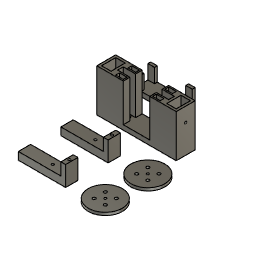
final v1 (Autodesk Fusion 360 design; units mm, degrees)
Autodesk Fusion 360 part; units mm, degrees
note: some values were not read from the file. Chosen so that the rebuilt part matches the saved one: which face or edge a step refers to; how an offset face is resized. Set by a fixed rule: which sketch regions a step uses.
sketch "Sketch1" plane through (0, 0, 0) normal (0, 0, 1) x (1, 0, 0)
  line L0 (0, 0) -> (84, 0)
  line L1 (84, 0) -> (84, 20)
  line L2 (84, 20) -> (0, 20)
  line L3 (0, 20) -> (0, 0)
  line L4 (0, 0) -> (0, 10)
  line L5 (0, 10) -> (84, 10) construction
  line L6 (42, 0) -> (42, 20) construction
  line L7 (42, 10) -> (60, 10) construction
  line L8 (42, 10) -> (24, 10) construction
  circle A0 centre (60, 10) radius 1.5
  circle A1 centre (24, 10) radius 1.5
  line L9 (79, 5) -> (79, 15)
  line L10 (5, 15) -> (5, 5)
  line L11 (5, 15) -> (10, 15)
  line L12 (10, 15) -> (10, 5)
  line L13 (79, 15) -> (74, 15)
  line L14 (74, 15) -> (74, 5)
  line L15 (79, 15) -> (74, 15)
  line L16 (10, 15) -> (5, 15)
  line L17 (5, 5) -> (10, 5)
  line L18 (74, 5) -> (79, 5)
  line L19 (0, 20) -> (15, 20)
  line L20 (15, 10) -> (15, 20)
  line L21 (84, 20) -> (69, 20)
  line L22 (69, 20) -> (69, 0)
  line L23 (15, 10) -> (15, 0)
  line L24 (12.5, 17.5) -> (2.5, 17.5)
  line L25 (2.5, 17.5) -> (2.5, 2.5)
  line L26 (2.5, 2.5) -> (12.5, 2.5)
  line L27 (12.5, 17.5) -> (12.5, 2.5)
  line L28 (71.5, 17.5) -> (71.5, 2.5)
  line L29 (71.5, 2.5) -> (81.5, 2.5)
  line L30 (81.5, 2.5) -> (81.5, 17.5)
  line L31 (81.5, 17.5) -> (71.5, 17.5)
  line L32 (0, 20) -> (0, 40) construction
  line L33 (0, 40) -> (47, 40)
  line L34 (47, 40) -> (47, 57)
  line L35 (47, 57) -> (0, 57)
  line L36 (0, 57) -> (0, 40)
  line L37 (0, 57) -> (7, 57)
  line L38 (7, 57) -> (7, 54)
  line L39 (7, 54) -> (0, 54)
  line L40 (0, 54) -> (0, 57)
  line L41 (0, 40) -> (0, 48.5)
  line L42 (47, 48.5) -> (0, 48.5)
  line L43 (0, 40) -> (7, 40)
  line L44 (7, 40) -> (7, 43)
  line L45 (7, 43) -> (0, 43)
  line L46 (0, 43) -> (0, 40)
  line L47 (47, 57) -> (40, 57)
  line L48 (40, 57) -> (40, 54)
  line L49 (40, 54) -> (47, 54)
  line L50 (47, 54) -> (47, 57)
  line L51 (47, 40) -> (40, 40)
  line L52 (40, 40) -> (40, 43)
  line L53 (40, 43) -> (47, 43)
  line L54 (47, 43) -> (47, 40)
  dimension "d1" = 84
  dimension "d2" = 20
  dimension "d6" = 3
  dimension "d7" = 3
  dimension "d9" = 5
  dimension "d10" = 5
  dimension "d31" = 2.5
  dimension "d32" = 2.5
  dimension "d96" = 47
  dimension "d97" = 17
  dimension "d98" = 3
  dimension "d99" = 7
  dimension "d100" = 3
  dimension "d101" = 7
  dimension "d102" = 3
  dimension "d103" = 7
  dimension "d104" = 3
  dimension "d105" = 7
  constraint coincident L0.start L3.end
  constraint horizontal L0
  constraint perpendicular L0 L1
  constraint perpendicular L1 L2
  constraint perpendicular L0 L3
  constraint midpoint L3 L4.end
  constraint midpoint L1 L5.end
  constraint midpoint L2 L6.end
  constraint perpendicular L2 L6
  constraint coincident L0 L6.start
  constraint midpoint L6 L7.start
  constraint perpendicular L6 L7
  constraint perpendicular L6 L8
  constraint coincident L7.end A0.centre
  constraint coincident L8.end A1.centre
  constraint perpendicular L10 L11
  constraint perpendicular L12 L17
  constraint perpendicular L9 L13
  constraint coincident L14.end L17
  constraint perpendicular L14 L17
  constraint collinear L15 L16
  constraint collinear L17 L18
  constraint coincident L2 L19.end
  constraint perpendicular L2 L20
  constraint coincident L2 L21.end
  constraint coincident L0 L22.end
  constraint perpendicular L0 L22
  constraint coincident L5 L20.start
  constraint coincident L0 L23.end
  constraint perpendicular L0 L23
  constraint perpendicular L19 L32
  constraint horizontal L33
  constraint vertical L34
  constraint horizontal L35
  constraint vertical L36
  constraint horizontal L37
  constraint vertical L38
  constraint horizontal L39
  constraint vertical L40
  constraint midpoint L36 L41.end
  constraint midpoint L34 L42.start
  constraint horizontal L43
  constraint vertical L44
  constraint horizontal L45
  constraint vertical L46
  constraint horizontal L47
  constraint vertical L48
  constraint horizontal L49
  constraint vertical L50
  constraint horizontal L51
  constraint vertical L52
  constraint horizontal L53
  constraint vertical L54
  measures "d1" distance of L0.start L0.end
  measures "d2" distance of L0.end L1.end
  measures "d6" diameter of A0
  measures "d7" diameter of A1
  measures "d9" distance of L10.start L11.end
  measures "d10" distance of L9.end L13.end
  measures "d96" distance of L32.end L33.end
  measures "d97" distance of L33.end L34.end
  measures "d98" distance of L37.end L38.end
  measures "d99" distance of L38.end L39.end
  measures "d100" distance of L43.end L44.end
  measures "d101" distance of L44.end L45.end
  measures "d102" distance of L47.end L48.end
  measures "d103" distance of L48.end L49.end
  measures "d104" distance of L51.end L52.end
  measures "d105" distance of L52.end L53.end
extrude "Extrude1" add sketch "Sketch1" along normal blind 5 contours L0 L2 L20 L22 L23 makes body 1
extrude "Extrude2" add sketch "Sketch1" along normal blind 45 contours L0 L2 L3 L4 L19 L20 L23 | L24 L25 L26 L27 bodies 1
extrude "Extrude3" add sketch "Sketch1" along normal blind 45 contours L0 L1 L2 L21 L22 | L28 L29 L30 L31 bodies 1
sketch "Sketch2" plane through (0, 0, 5) normal (0, 0, 1) x (-1, 0, 0)
  circle A0 centre (-24, -10) radius 1.5
  circle A1 centre (-60, -10) radius 1.5
  line L0 (-69, -20) -> (-15, -20)
  line L1 (-15, -20) -> (-15, 0)
  line L2 (-15, 0) -> (-69, 0)
  line L3 (-69, 0) -> (-69, -20)
  line L4 (-42, -10) -> (-56, -10)
  line L5 (-56, -13) -> (-56, -20)
  line L6 (-56, -7) -> (-56, 0)
  line L7 (-42, -10) -> (-28, -10)
  line L8 (-28, -7) -> (-28, 0)
  line L9 (-28, -13) -> (-28, -20)
  line L10 (-26, -13) -> (-26, -20)
  line L11 (-26, -7) -> (-26, 0)
  line L12 (-58, -13) -> (-58, -20)
  line L13 (-58, -7) -> (-58, 0)
  line L14 (-26, -20) -> (-26, -13)
  line L15 (-26, -20) -> (-26, -13)
  line L16 (-28, -13) -> (-26, -13)
  line L17 (-56, -20) -> (-56, -13)
  line L18 (-58, -13) -> (-56, -13)
  line L19 (-26, 0) -> (-26, -7)
  line L20 (-28, -7) -> (-26, -7)
  line L21 (-56, 0) -> (-56, -7)
  line L22 (-58, -7) -> (-56, -7)
  dimension "d18" = -2
  dimension "d20" = 2
  dimension "d22" = 14
  constraint horizontal L4
  constraint coincident L0 L5.end
  constraint perpendicular L0 L5
  constraint coincident L2 L6.end
  constraint perpendicular L2 L6
  constraint parallel L4 L7
  constraint coincident L2 L8.end
  constraint perpendicular L2 L8
  constraint coincident L0 L9.end
  constraint perpendicular L0 L9
  constraint coincident L10 L14.end
  constraint perpendicular L7 L14
  constraint perpendicular L15 L16
  constraint coincident L12 L18.start
  constraint perpendicular L5 L18
  constraint perpendicular L19 L20
  constraint perpendicular L6 L22
  measures "d22" distance of L4.start L7.end
extrude "Extrude4" add sketch "Sketch2" along normal blind 14 contours L0 L9 L10 L14 L15 L16 bodies 1
extrude "Extrude5" cut 1 faces at (27.3333, 15.3333, 19) along direction (0, 0, -1) blind 14 on bodies 1 bodies 1
extrude "Extrude6" cut 1 faces at (36.1113, 2.8459, 0) along direction (0, 0, -1) blind 14 on bodies 1 bodies 1
extrude "Extrude7" add sketch "Sketch2" along normal blind 20 contours L0 L5 L12 L17 L18 | L2 L6 L13 L21 L22 | L0 L9 L10 L14 L15 L16 | L2 L8 L11 L19 L20 bodies 1
extrude "Extrude8" cut sketch "Sketch1" along normal blind 55 contours L24 L25 L26 L27 bodies 1
extrude "Extrude9" cut sketch "Sketch1" along normal blind 53 contours L28 L29 L30 L31 bodies 1
sketch "Sketch4" plane through (0, 0, 0) normal (1, 0, 0) x (0, 1, 0)
  line L0 (0, 0) -> (-20, 0) construction
  line L1 (-20, 0) -> (-28, 0)
  line L2 (-28, 0) -> (-28, 13)
  line L3 (-28, 13) -> (-20, 13)
  line L4 (-20, 13) -> (-20, 0)
  dimension "d40" = 20
  dimension "d41" = 8
  dimension "d42" = 13
  constraint coincident L0.start origin
  constraint horizontal L0
  constraint horizontal L1
  constraint vertical L2
  constraint horizontal L3
  constraint vertical L4
  measures "d40" distance of L0.start L0.end
  measures "d41" distance of L0.end L1.end
  measures "d42" distance of L1.end L2.end
extrude "Extrude10" add sketch "Sketch4" along normal blind 50 separate body makes body 2
sketch "Sketch5" plane through (0, -28, 0) normal (0, -1, 0) x (1, 0, 0)
  line L0 (0, 13) -> (0, 0)
  line L1 (0, 0) -> (50, 0)
  line L2 (50, 0) -> (50, 13)
  line L3 (50, 13) -> (0, 13)
  line L4 (50, 13) -> (45, 13)
  line L5 (45, 13) -> (45, 0)
  dimension "d45" = 5
  constraint coincident L2.end L3.start
  constraint perpendicular L2 L4
  constraint coincident L1 L5.end
  constraint perpendicular L1 L5
  measures "d45" distance of L2.end L4.end
extrude "Extrude11" add sketch "Sketch5" along normal blind 15 contours L1 L2 L3 L4 L5 bodies 2
sketch "Sketch6" plane through (0, 0, 0) normal (0, 0, 1) x (1, 0, 0)
  circle A0 centre (84, -30) radius 18
  line L0 (88.7553, -25.2447) -> (89.8867, -24.1133)
  line L1 (88.7553, -34.7553) -> (89.8867, -35.8867)
  line L2 (79.2447, -25.2447) -> (78.1133, -24.1133)
  line L3 (79.2447, -34.7553) -> (78.1133, -35.8867)
  circle A1 centre (89.8867, -24.1133) radius 1.6
  circle A2 centre (78.1133, -24.1133) radius 1.6
  circle A3 centre (89.8867, -35.8867) radius 1.6
  circle A4 centre (78.1133, -35.8867) radius 1.6
  arc A5 (79.3482, -23.0959) -> (77.0959, -25.3482) centre (84, -30) ccw
  arc A6 (77.0959, -34.6518) -> (78.1133, -35.8867) centre (84, -30) ccw
  arc A7 (88.6518, -36.9041) -> (90.9041, -34.6518) centre (84, -30) ccw
  arc A8 (90.9041, -25.3482) -> (88.6518, -23.0959) centre (84, -30) ccw
  circle A9 centre (84, -30) radius 1.5
  dimension "d49" = 36
  dimension "d50" = 16.65
  dimension "d51" = 3.2
  dimension "d52" = 3.2
  dimension "d53" = 3.2
  dimension "d54" = 3.2
  dimension "d57" = 3
  constraint concentric A0 A5
  constraint coincident L1.end A5
  constraint perpendicular L0 L1
  constraint perpendicular L0 L2
  constraint perpendicular L2 L3
  constraint coincident L3.end A5
  constraint coincident L0.end A5
  constraint coincident L2.end A5
  constraint coincident L0.end A1.centre
  constraint coincident L2.end A2.centre
  constraint coincident L1.end A3.centre
  constraint coincident L3.end A4.centre
  constraint coincident A1 A8.end
  constraint coincident A2 A5.start
  constraint coincident A2 A5.end
  constraint coincident A4 A6.start
  constraint concentric A5 A6
  constraint concentric A6 A7
  constraint coincident A3 A7.start
  constraint coincident A3 A7.end
  constraint coincident A1 A8.start
  constraint concentric A7 A8
  constraint coincident A3 L1.start
  constraint coincident A4 L3.start
  constraint coincident A1 L0.start
  constraint coincident A2 L2.start
  constraint concentric A6 A9
  measures "d49" diameter of A0
  measures "d50" diameter of A5
  measures "d51" diameter of A1
  measures "d52" diameter of A2
  measures "d53" diameter of A3
  measures "d54" diameter of A4
  measures "d57" diameter of A9
extrude "Extrude12" add sketch "Sketch6" along normal blind 3 separate body contours A0 | A9 makes body 3
sketch "Sketch7" plane through (0, 0, 3) normal (0, 0, 1) x (-1, 0, 0)
  circle A0 centre (-78.1133, 35.8867) radius 1.6
  circle A1 centre (-89.8867, 35.8867) radius 1.6
  circle A2 centre (-78.1133, 24.1133) radius 1.6
  circle A3 centre (-89.8867, 24.1133) radius 1.6
  circle A4 centre (-84, 30) radius 18
  circle A5 centre (-84, 30) radius 1.5
  dimension "d58" = 3
  constraint concentric A4 A5
  measures "d58" diameter of A5
extrude "Extrude13" cut sketch "Sketch7" against normal blind 11 contours A5 bodies 3
thread "Thread1" "ISO Metric profile 3.0 M3x0.5 6H" major diameter 3.086 minor diameter 2.529 pitch 0.5 angle 60 resizes the face on face at (82.8043, -30.9057, 1) on bodies 3
sketch "Sketch8" plane through (0, -43, 0) normal (0, -1, 0) x (1, 0, 0)
  line L0 (45, 13) -> (45, 0)
  line L1 (45, 0) -> (50, 0)
  line L2 (50, 0) -> (50, 13)
  line L3 (50, 13) -> (45, 13)
  circle A0 centre (47.5, 6.5) radius 1.5
  dimension "d61" = 3
  measures "d61" diameter of A0
extrude "Extrude14" cut sketch "Sketch8" against normal blind 27 contours A0 bodies 2
extrude "Extrude15" cut 1 faces at (47.5374, -43, 1.6681) along direction (0, 1, 0) blind 2 on bodies 2 bodies 2
sketch "Sketch10" plane through (0, 0, 0) normal (1, 0, 0) x (0, 1, 0)
  line L0 (-28, 0) -> (-38, 0) construction
  line L1 (-38, 0) -> (-88, 0)
  dimension "d66" = 10
  dimension "d79" = 50
  constraint horizontal L0
  constraint parallel L0 L1
  measures "d66" distance of L0.start L0.end
  measures "d79" distance of L0.end L1.end
move_body "Move1" bodies 2 to x (1, 0, 0) y (0, 1, 0) z (0, 0, 1) at (0, -18, 0)
move_body "Move2" bodies 2 to x (1, 0, 0) y (0, 0, -1) z (0, 1, 0) at (0, -38, -38)
thread "Thread2" "ISO Metric profile 3.0 M3x0.5 6H" major diameter 3.086 minor diameter 2.529 pitch 0.5 angle 60 resizes the face on face at (47.9063, -30.0561, 14) on bodies 2
sketch "Sketch11" plane through (0, 0, 8) normal (0, 0, 1) x (-1, 0, 0)
  line L0 (-45, 38) -> (-45, 25)
  line L1 (-45, 25) -> (0, 25)
  line L2 (0, 25) -> (0, 38)
  line L3 (0, 38) -> (-45, 38)
  line L4 (0, 25) -> (0, 31.5)
  circle A0 centre (-30, 31.5) radius 1.5
  dimension "d68" = 3
  constraint coincident L1.end L2.start
  constraint midpoint L2 L4.end
  measures "d68" diameter of A0
extrude "Extrude16" cut sketch "Sketch11" against normal blind 18 contours A0 bodies 2
thread "Thread3" "ISO Metric profile 3.0 M3x0.5 6H" major diameter 3.086 minor diameter 2.529 pitch 0.5 angle 60 resizes the face on face at (29.1244, -32.7179, 2.6667) on bodies 2
sketch "Sketch12" plane through (0, 0, 0) normal (-1, 0, 0) x (0, -1, 0)
  line L0 (-20, 0) -> (0, 0)
  line L1 (0, 0) -> (0, 45)
  line L2 (0, 45) -> (-20, 45)
  line L3 (-20, 45) -> (-20, 0)
  line L4 (-20, 45) -> (-10, 45)
  line L5 (-10, 45) -> (-10, 30)
  circle A0 centre (-10, 30) radius 1.5
  dimension "d71" = 15
  dimension "d72" = 3
  constraint coincident L2.end L3.start
  constraint midpoint L2 L4.end
  constraint perpendicular L4 L5
  constraint coincident L5.end A0.centre
  measures "d71" distance of L4.end L5.end
  measures "d72" diameter of A0
extrude "Extrude17" cut sketch "Sketch12" against normal blind 33 contours A0 bodies 1
thread "Thread4" "ISO Metric profile 3.0 M3x0.5 6H" major diameter 3.086 minor diameter 2.529 pitch 0.5 angle 60 resizes the face on face at (0.8333, 8.5075, 30.1494) on bodies 1
thread "Thread5" "ISO Metric profile 3.0 M3x0.5 6H" major diameter 3.086 minor diameter 2.529 pitch 0.5 angle 60 resizes the face on face at (14.1667, 11.4925, 29.8506) on bodies 1
sketch "Sketch13" plane through (84, 0, 0) normal (1, 0, 0) x (0, 1, 0)
  line L0 (0, 0) -> (20, 0)
  line L1 (20, 0) -> (20, 45)
  line L2 (20, 45) -> (0, 45)
  line L3 (0, 45) -> (0, 0)
  line L4 (10, 45) -> (10, 30)
  circle A0 centre (10, 30) radius 1.5
  dimension "d75" = 15
  dimension "d76" = 3
  constraint midpoint L2 L4.start
  constraint perpendicular L2 L4
  constraint coincident L4.end A0.centre
  measures "d75" distance of L4.start L4.end
  measures "d76" diameter of A0
extrude "Extrude18" cut sketch "Sketch13" against normal blind 31 contours A0 bodies 1
thread "Thread6" "ISO Metric profile 3.0 M3x0.5 6H" major diameter 3.086 minor diameter 2.529 pitch 0.5 angle 60 resizes the face on face at (83.1667, 11.4925, 30.1494) on bodies 1
thread "Thread7" "ISO Metric profile 3.0 M3x0.5 6H" major diameter 3.086 minor diameter 2.529 pitch 0.5 angle 60 resizes the face on face at (69.8333, 11.4925, 29.8506) on bodies 1
copy_body "CopyPasteBodies1" bodies 2 3 makes body 4 makes body 5
move_body "Move3" bodies 4 5 to x (1, 0, 0) y (0, 1, 0) z (0, 0, 1) at (0, -45, 0)
sketch "Sketch14" plane through (0, 0, 5) normal (0, 0, 1) x (-1, 0, 0)
  line L0 (-56, -13) -> (-56, -20)
  line L1 (-56, -20) -> (-28, -20)
  line L2 (-28, -20) -> (-28, -13)
  line L3 (-28, -13) -> (-26, -13)
  line L4 (-26, -13) -> (-26, -20)
  line L5 (-26, -20) -> (-15, -20)
  line L6 (-15, -20) -> (-15, 0)
  line L7 (-15, 0) -> (-26, 0)
  line L8 (-26, 0) -> (-26, -7)
  line L9 (-26, -7) -> (-28, -7)
  line L10 (-28, -7) -> (-28, 0)
  line L11 (-28, 0) -> (-56, 0)
  line L12 (-56, 0) -> (-56, -7)
  line L13 (-56, -7) -> (-58, -7)
  line L14 (-58, -7) -> (-58, 0)
  line L15 (-58, 0) -> (-69, 0)
  line L16 (-69, 0) -> (-69, -20)
  line L17 (-69, -20) -> (-58, -20)
  line L18 (-58, -20) -> (-58, -13)
  line L19 (-58, -13) -> (-56, -13)
  circle A0 centre (-60, -10) radius 1.5
  circle A1 centre (-24, -10) radius 1.5
  line L20 (-28, 0) -> (-15, 0)
  line L21 (-15, 0) -> (-15, -7)
  line L22 (-15, -7) -> (-28, -7)
  line L23 (-28, -7) -> (-28, 0)
  line L24 (-28, -13) -> (-15, -13)
  line L25 (-15, -13) -> (-15, -20)
  line L26 (-15, -20) -> (-28, -20)
  line L27 (-28, -20) -> (-28, -13)
  line L28 (-56, -20) -> (-69, -20)
  line L29 (-69, -20) -> (-69, -13)
  line L30 (-69, -13) -> (-56, -13)
  line L31 (-56, -13) -> (-56, -20)
  line L32 (-56, -7) -> (-69, -7)
  line L33 (-69, -7) -> (-69, 0)
  line L34 (-69, 0) -> (-56, 0)
  line L35 (-56, 0) -> (-56, -7)
  constraint horizontal L20
  constraint vertical L21
  constraint horizontal L22
  constraint vertical L23
  constraint coincident L6 L21.end
  constraint coincident L10.end L11.start
  constraint horizontal L24
  constraint vertical L25
  constraint horizontal L26
  constraint vertical L27
  constraint coincident L5.end L6.start
  constraint coincident L2.end L3.start
  constraint horizontal L28
  constraint vertical L29
  constraint horizontal L30
  constraint vertical L31
  constraint coincident L16 L29.end
  constraint coincident L0.end L1.start
  constraint horizontal L32
  constraint vertical L33
  constraint horizontal L34
  constraint vertical L35
  constraint coincident L15.end L16.start
  constraint coincident L12.end L13.start
extrude "Extrude19" add sketch "Sketch14" along normal blind 40 contours L6 L7 L8 L20 L21 L22 bodies 1
extrude "Extrude20" add 4 faces at (27.3333, 2.3333, 25) (57.3333, 2.3333, 25) (56.6667, 17.6667, 25) (26.6667, 17.6667, 25) along direction (0, 0, 1) blind 20 on bodies 1 bodies 1
extrude "Extrude21" add sketch "Sketch14" along normal blind 40 contours L16 L17 L18 L28 L29 L30 | L4 L5 L6 L24 L25 L26 | L14 L15 L16 L32 L33 L34 bodies 1
sketch "Sketch15" plane through (0, 0, 45) normal (0, 0, 1) x (-1, 0, 0)
  line L0 (-2.5, -17.5) -> (-12.5, -17.5)
  line L1 (-12.5, -17.5) -> (-12.5, -2.5)
  line L2 (-12.5, -2.5) -> (-2.5, -2.5)
  line L3 (-2.5, -2.5) -> (-2.5, -17.5)
  line L4 (-28, -20) -> (0, -20)
  line L5 (0, -20) -> (0, 0)
  line L6 (0, 0) -> (-28, 0)
  line L7 (-28, 0) -> (-28, -7)
  line L8 (-28, -7) -> (-15, -7)
  line L9 (-15, -7) -> (-15, -13)
  line L10 (-15, -13) -> (-28, -13)
  line L11 (-28, -13) -> (-28, -20)
  line L12 (-18.5, -1.5) -> (-26.5, -1.5)
  line L13 (-26.5, -1.5) -> (-26.5, -5.5)
  line L14 (-26.5, -5.5) -> (-18.5, -5.5)
  line L15 (-18.5, -14.5) -> (-26.5, -14.5)
  line L16 (-26.5, -14.5) -> (-26.5, -18.5)
  line L17 (-26.5, -18.5) -> (-18.5, -18.5)
  line L18 (-1.5, -18.5) -> (-1.5, -1.5)
  line L19 (-26.5, -14.5) -> (-18.5, -14.5)
  line L20 (-18.5, -14.5) -> (-18.5, -18.5)
  line L21 (-18.5, -18.5) -> (-26.5, -18.5)
  line L22 (-26.5, -18.5) -> (-26.5, -14.5)
  line L23 (-26.5, -1.5) -> (-18.5, -1.5)
  line L24 (-18.5, -1.5) -> (-18.5, -5.5)
  line L25 (-18.5, -5.5) -> (-26.5, -5.5)
  line L26 (-26.5, -5.5) -> (-26.5, -1.5)
  dimension "d87" = 8
  dimension "d88" = 8
  constraint horizontal L19
  constraint vertical L20
  constraint horizontal L21
  constraint vertical L22
  constraint horizontal L23
  constraint vertical L24
  constraint horizontal L25
  constraint vertical L26
  measures "d87" distance of L15.end L15.start
  measures "d88" distance of L12.end L12.start
extrude "Extrude22" cut sketch "Sketch15" against normal blind 49 contours L12 L13 L14 L23 L24 L25 L26 | L15 L16 L17 L19 L20 L21 L22 bodies 1
sketch "Sketch16" plane through (0, 0, 45) normal (0, 0, 1) x (-1, 0, 0)
  line L0 (-81.5, -17.5) -> (-81.5, -2.5)
  line L1 (-81.5, -2.5) -> (-71.5, -2.5)
  line L2 (-71.5, -2.5) -> (-71.5, -17.5)
  line L3 (-71.5, -17.5) -> (-81.5, -17.5)
  line L4 (-69, -13) -> (-69, -7)
  line L5 (-69, -7) -> (-56, -7)
  line L6 (-56, -7) -> (-56, 0)
  line L7 (-56, 0) -> (-84, 0)
  line L8 (-84, 0) -> (-84, -20)
  line L9 (-84, -20) -> (-56, -20)
  line L10 (-56, -20) -> (-56, -13)
  line L11 (-56, -13) -> (-69, -13)
  line L12 (-57.5, -14.5) -> (-65.5, -14.5)
  line L13 (-65.5, -5.5) -> (-57.5, -5.5)
  line L14 (-57.5, -5.5) -> (-57.5, -1.5)
  line L15 (-57.5, -1.5) -> (-65.5, -1.5)
  line L16 (-65.5, -18.5) -> (-57.5, -18.5)
  line L17 (-57.5, -18.5) -> (-57.5, -14.5)
  line L18 (-57.5, -18.5) -> (-65.5, -18.5)
  line L19 (-65.5, -18.5) -> (-65.5, -14.5)
  line L20 (-65.5, -14.5) -> (-57.5, -14.5)
  line L21 (-57.5, -14.5) -> (-57.5, -18.5)
  line L22 (-57.5, -5.5) -> (-65.5, -5.5)
  line L23 (-65.5, -5.5) -> (-65.5, -1.5)
  line L24 (-65.5, -1.5) -> (-57.5, -1.5)
  line L25 (-57.5, -1.5) -> (-57.5, -5.5)
  dimension "d92" = 8
  dimension "d93" = 8
  constraint horizontal L18
  constraint vertical L19
  constraint horizontal L20
  constraint vertical L21
  constraint horizontal L22
  constraint vertical L23
  constraint horizontal L24
  constraint vertical L25
  measures "d92" distance of L16.end L16.start
  measures "d93" distance of L13.end L13.start
extrude "Extrude23" cut sketch "Sketch16" against normal blind 56 contours L12 L16 L17 L18 L19 L20 L21 | L13 L14 L15 L22 L23 L24 L25 bodies 1
extrude "Extrude24" add sketch "Sketch1" along normal blind 5 separate body contours L33 L34 L36 L41 L42 L44 L45 L52 L53 | L34 L35 L36 L38 L39 L42 L48 L49 makes body 6
extrude "Extrude25" add sketch "Sketch1" along normal blind 20 contours L33 L36 L41 L43 L44 L45 L46 | L33 L34 L51 L52 L53 L54 | L35 L36 L37 L38 L39 L40 | L34 L35 L47 L48 L49 L50 bodies 6
